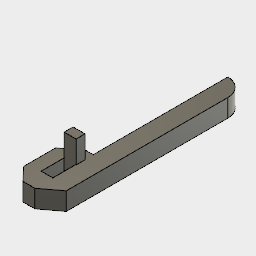
四轴护罩部件02 (Autodesk Fusion 360 design; units mm, degrees)
Autodesk Fusion 360 part; units mm, degrees
sketch "草图1" plane through (0, 0, 0) normal (0, 1, 0) x (1, 0, 0)
  line L0 (0, 0) -> (4, 0)
  line L1 (4, 0) -> (4, 35)
  line L2 (4, 35) -> (0, 35)
  line L3 (0, 35) -> (0, 0)
  line L4 (4, 0) -> (-5.5, 0)
  line L5 (-5.5, 0) -> (-5.5, -4)
  line L6 (-5.5, -4) -> (4, -4)
  line L7 (4, -4) -> (4, 0)
  line L8 (-5.5, 0) -> (-2.6, 0)
  line L9 (-2.6, 0) -> (-2.6, 9)
  line L10 (-2.6, 9) -> (-5.5, 9)
  line L11 (-5.5, 9) -> (-5.5, 0)
  line L12 (-2.6, 9) -> (0, 9)
  line L13 (0, 9) -> (0, 5.1)
  line L14 (0, 5.1) -> (-2.6, 5.1)
  line L15 (-2.6, 5.1) -> (-2.6, 9)
  arc A0 (4, 35) -> (0, 39) centre (0, 35) ccw
  line L16 (0, 39) -> (0, 35)
  dimension "d1" = 35
  dimension "d2" = 4
  dimension "d3" = 4
  dimension "d4" = 9.5
  dimension "d5" = 9
  dimension "d6" = 3.9
  dimension "d11" = 2.9
  measures "d1" distance of L0.start L2.end
  measures "d2" distance of L1.end L2.end
  measures "d3" distance of L0.end L6.end
  measures "d4" distance of L0.end L4.end
  measures "d5" distance of L4.end L10.end
  measures "d6" distance of L9.end L14.end
  measures "d11" distance of L4.end L8.end
extrude "拉伸1" add sketch "草图1" along normal blind 3 contours L0 L1 L2 L3 L4 L13 | L0 L4 L5 L6 L7 L8 | L3 L9 L12 L13 L14 L15 | L4 L8 L9 L10 L11 L15
extrude "拉伸2" cut 1 faces at (2.6667, 3, -14.6667) along direction (0, -1, 0) blind 3
extrude "拉伸3" add sketch "草图1" along normal blind 4 contours L0 L1 L2 L3 L4 L13 | L0 L4 L5 L6 L7 L8 | L3 L9 L12 L13 L14 L15 | L4 L8 L9 L10 L11 L15 | L2 A0 L16
sketch "草图2" plane through (0, 4, 0) normal (0, 1, 0) x (-1, 0, 0)
  line L0 (0, -5.1) -> (0, 0)
  line L1 (0, 0) -> (2.6, 0)
  line L2 (2.6, 0) -> (2.6, -5.1)
  line L3 (2.6, -5.1) -> (0, -5.1)
  line L4 (0, -9) -> (5.5, -9)
  line L5 (5.5, -9) -> (5.5, 4)
  line L6 (5.5, 4) -> (-4, 4)
  line L7 (-4, 4) -> (-4, -35)
  arc A0 (-4, -35) -> (0, -39) centre (0, -35) ccw
  line L8 (0, -39) -> (0, -9)
  line L9 (2.6, -5.1) -> (-0.1, -5.1)
  line L10 (-0.1, -5.1) -> (-0.1, -7.1)
  line L11 (-0.1, -7.1) -> (2.6, -7.1)
  line L12 (2.6, -7.1) -> (2.6, -5.1)
  line L13 (5.5, 1) -> (2.7, 4)
  line L14 (0, 4) -> (-4, 1)
  line L15 (5.5, -6.1253) -> (1.6475, -9)
  dimension "d14" = 2
  measures "d14" distance of L2.end L11.end
extrude "拉伸4" add sketch "草图2" along normal blind 4 contours L3 L9 L10 L11 L12
extrude "拉伸5" add 1 faces at (-0.8, 8, -5.7667) along direction (0, 1, 0) blind 1
extrude "拉伸6" cut sketch "草图2" against normal blind 5 contours L4 L5 L15 | L5 L6 L13 | L6 L7 L14
